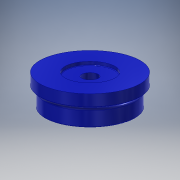
# Autodesk Inventor part: Component 42(Minehmer)
Saved by Autodesk Inventor 2018 (Build 220112000, 112)
## iProperties
Created: 2023-04-01
Part Number: Component 42(Minehmer)
Material: Generic
Document SubType Name: Modeling
Designer: Habib Mohamed
Density: 1 g/cm^3
Appearance: Blue - Wall Paint - Glossy
Author: Habib Mohamed
Autodesk Inventor part; units mm, degrees
ref_plane "YZ Plane" through (0, 0, 0) normal (1, 0, 0) x (0, 1, 0)
ref_plane "XZ Plane" through (0, 0, 0) normal (0, 1, 0) x (-1, 0, 0)
ref_plane "XY Plane" through (0, 0, 0) normal (0, 0, 1) x (1, 0, 0)
sketch "Sketch1" plane through (0, 0, 0) normal (1, 0, 0) x (0, 1, 0)
  line L0 (12.9, -10) -> (12.9, -20)
  line L1 (12.9, -20) -> (8.2361, -20)
  line L2 (8, -20) -> (8, -20)
  line L3 (6, -18) -> (0.25, -18)
  line L4 (0, -17.75) -> (0, -6.0156)
  line L5 (0.198, -5.7711) -> (11.4, -3.39)
  line L6 (11.4, -3.39) -> (11.4, -9.75)
  line L7 (11.65, -10) -> (12.9, -10)
  arc A0 (11.4, -9.75) -> (11.65, -10) centre (11.65, -9.75) ccw
  arc A1 (0.198, -5.7711) -> (0, -6.0156) centre (0.25, -6.0156) ccw
  arc A2 (0, -17.75) -> (0.25, -18) centre (0.25, -17.75) ccw
  arc A3 (7.9876, -19.7778) -> (6, -18) centre (6, -20) ccw
  arc A4 (7.9876, -19.7778) -> (8.2361, -20) centre (8.2361, -19.75) ccw
  line L8 (0, 0) -> (26.0527, 0) construction
  point P0 (11.4, -10)
  dimension "d0" = 10
  dimension "d1" = 12.9
  dimension "d2" = 8
  dimension "d3" = 20
  dimension "d4" = 18
  dimension "d5" = 1.5
  dimension "d6" = 3.39
  dimension "d7" = 78
  dimension "d8" = 12.9
  dimension "d9" = 0.25
  dimension "d10" = 2
  dimension "d11" = 0.25
  constraints: 18 end point, 11 point on circle, 10 tangent, 5 centre point, 5 perpendicular, 3 point on line, 2 equal radius, 1 horizontal, 1 parallel, 1 vertical
  measures "d0" distance from line of L7 L8.start
  measures "d1" distance between parallel lines of L0 L4
  measures "d2" distance between parallel lines of L4 L2
  measures "d3" distance from line of L8.start L1
  measures "d4" distance from line of L8.start L3
  measures "d5" distance of point (11.4, -10) L0.start
  measures "d6" vertical distance of L8.start L5.end
  measures "d7" angle of L5 L6
  measures "d8" distance from line of L0 L8.start
  measures "d9" radius of A0
  measures "d10" radius of A3
  measures "d11" radius of A4
revolve "Revolution1" add sketch "Sketch1" angle 360 about axis through (0, 0, 0) along (0, 1, 0)
body "Solid1"
